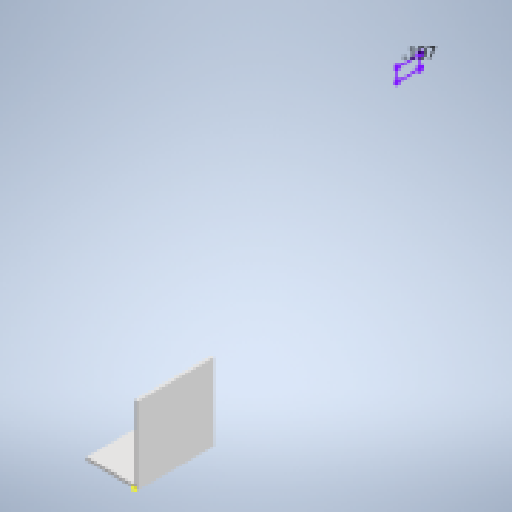
# Autodesk Inventor part: BK10_Z_Mount
Saved by Autodesk Inventor 2023 (Build 270158000, 158)
## iProperties
Created: 2022-05-07
Part Number: BK10_Z_Mount
Material: Generic
Document SubType Name: Modeling
Designer: plebbb
Density: 1 g/cm^3
Appearance: Default
Mass: 29.9576 g
Surface Area: 201.411 cm^2
Volume: 29.9576 cm^3
Author: plebbb
Autodesk Inventor part; units mm, degrees
ref_plane "YZ Plane" through (0, 0, 0) normal (1, 0, 0) x (0, 1, 0)
ref_plane "XZ Plane" through (0, 0, 0) normal (0, 1, 0) x (-1, 0, 0)
ref_plane "XY Plane" through (0, 0, 0) normal (0, 0, 1) x (1, 0, 0)
sketch "Sketch1" plane through (0, 0, 0) normal (0, 1, 0) x (-1, 0, 0)
  line L0 (0, 0) -> (50.8, 0)
  line L1 (50.8, 0) -> (50.8, -76.2)
  line L2 (50.8, -76.2) -> (0, -76.2)
  line L3 (0, -76.2) -> (0, 0)
  dimension "d0" = 50.8
  dimension "d1" = 76.2
  constraints: 8 end point, 2 parallel, 1 horizontal, 1 perpendicular
  measures "d0" distance of L1.end L2.end
  measures "d1" distance of L0.end L1.end
extrude "Extrusion1" add sketch "Sketch1" along normal blind 76.2
shell "Shell1" thickness 3.175 removed faces 4 at (-33.8667, 25.4, 0) at (-50.8, 25.4, -50.8) at (-16.9333, 25.4, -76.2) at (-33.8667, 76.2, -50.8)
sketch "Sketch2" plane through (-3.175, 3.175, 0) normal (-1, 0, 0) x (0, 0, 1)
  circle A0 centre (-15.1, 40.925) radius 2.5
  circle A1 centre (-61.1, 53.925) radius 2.5
  circle A2 centre (-61.1, 40.925) radius 2.5
  circle A3 centre (-15.1, 53.925) radius 2.5
  line L0 (-61.1, 53.925) -> (-15.1, 53.925) construction
  line L1 (-15.1, 53.925) -> (-15.1, 40.925) construction
  line L2 (-15.1, 40.925) -> (-61.1, 40.925) construction
  line L3 (-61.1, 40.925) -> (-61.1, 53.925) construction
  line L4 (0, 0) -> (-76.2, 0) projected
  point P0 (0, -3.175)
  point P1 (-38.1, 53.925)
  point P2 (-38.1, 0)
  dimension "d5" = 5
  dimension "d6" = 46
  dimension "d7" = 13
  dimension "d8" = 40.925
  constraints: 8 end point, 4 centre point, 4 coincident, 3 equal radius, 2 midpoint, 2 parallel, 1 horizontal, 1 perpendicular, 1 vertical alignment
  measures "d5" diameter of A1
  measures "d6" distance of L0.start L0.end
  measures "d7" distance of L0.end L1.end
  measures "d8" distance between parallel lines of L4 L2
extrude "Extrusion2" cut sketch "Sketch2" against normal blind 25.4
body "Solid1"
